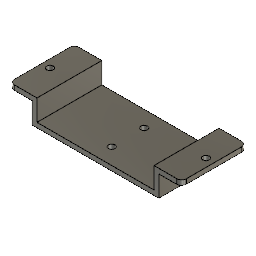
Chasis Quadra v19 (Autodesk Fusion 360 archive; units mm, degrees)
design "Soporte baterias"
Autodesk Fusion 360 part; units mm, degrees
sketch "Sketch1" plane through (0, 0, 0) normal (0, 0, 1) x (1, 0, 0)
  line L0 (0, 0) -> (78, 0)
  line L1 (78, 0) -> (78, 40)
  line L2 (78, 40) -> (0, 40)
  line L3 (0, 40) -> (0, 0)
  dimension "d1" = 78
  dimension "d2" = 40
  constraint horizontal L0
  constraint vertical L1
  constraint horizontal L2
  constraint vertical L3
  constraint coincident L0.start L3.end
  measures "d1" distance of L1.end L2.end
  measures "d2" distance of L0.start L2.end
extrude "Extrude1" add sketch "Sketch1" along normal blind 3
sketch "Sketch3" plane through (0, 0, 3) normal (0, 0, 1) x (-1, 0, 0)
  line L0 (0, -40) -> (0, 0)
  line L1 (0, 0) -> (-78, 0)
  line L2 (-78, 0) -> (-78, -40)
  line L3 (-78, -40) -> (0, -40)
  line L4 (0, -40) -> (-3, -40)
  line L5 (-3, -40) -> (-3, 0)
  line L6 (0, 0) -> (0, -40)
  dimension "d5" = 3
  constraint coincident L0.start L3.end
  constraint perpendicular L0 L4
  constraint coincident L1 L5.end
  constraint perpendicular L1 L5
  constraint coincident L0.end L1.start
  measures "d5" distance of L0.start L4.end
extrude "Extrude2" add sketch "Sketch3" along normal blind 13 contours L0 L1 L3 L4 L5 L6
sketch "Sketch4" plane through (0, 0, 3) normal (0, 0, 1) x (-1, 0, 0)
  line L0 (-3, -40) -> (-3, 0)
  line L1 (-3, 0) -> (-78, 0)
  line L2 (-78, 0) -> (-78, -40)
  line L3 (-78, -40) -> (-3, -40)
  line L4 (-78, -40) -> (-75, -40)
  line L5 (-75, -40) -> (-75, 0)
  line L6 (-78, 0) -> (-78, -40)
  dimension "d8" = 3
  constraint coincident L2.end L3.start
  constraint perpendicular L2 L4
  constraint coincident L1 L5.end
  constraint perpendicular L1 L5
  constraint coincident L1.end L2.start
  measures "d8" distance of L2.end L4.end
extrude "Extrude3" add sketch "Sketch4" along normal blind 13 contours L1 L2 L3 L4 L5 L6
sketch "Sketch5" plane through (78, 0, 0) normal (1, 0, 0) x (0, 1, 0)
  line L0 (0, 0) -> (40, 0)
  line L1 (40, 0) -> (40, 16)
  line L2 (40, 16) -> (0, 16)
  line L3 (0, 16) -> (0, 0)
  line L4 (40, 16) -> (40, 13)
  line L5 (40, 13) -> (0, 13)
  line L6 (0, 13) -> (0, 16)
  constraint coincident L1.end L2.start
  constraint coincident L1 L4.end
  constraint perpendicular L2 L4
  constraint coincident L3 L5.end
  constraint perpendicular L3 L5
  constraint coincident L2.end L3.start
  constraint perpendicular L2 L6
extrude "Extrude4" add sketch "Sketch5" along normal blind 14 contours L1 L2 L3 L4 L5 L6
sketch "Sketch6" plane through (0, 0, 0) normal (-1, 0, 0) x (0, -1, 0)
  line L0 (-40, 0) -> (0, 0)
  line L1 (0, 0) -> (0, 16)
  line L2 (0, 16) -> (-40, 16)
  line L3 (-40, 16) -> (-40, 0)
  line L4 (-40, 16) -> (0, 16)
  line L5 (0, 16) -> (0, 13)
  line L6 (0, 13) -> (-40, 13)
  line L7 (-40, 13) -> (-40, 16)
  constraint coincident L2.end L3.start
  constraint coincident L1.end L2.start
  constraint coincident L1 L5.end
  constraint perpendicular L4 L5
  constraint coincident L3 L6.end
  constraint perpendicular L3 L6
  constraint perpendicular L2 L7
extrude "Extrude5" add sketch "Sketch6" along normal blind 14 contours L1 L2 L3 L4 L5 L6 L7
sketch "Sketch7" plane through (0, 0, 16) normal (0, 0, 1) x (-1, 0, 0)
  line L0 (14, 0) -> (-3, 0)
  line L1 (-3, 0) -> (-3, -40)
  line L2 (-3, -40) -> (14, -40)
  line L3 (14, -40) -> (14, 0)
  circle A0 centre (9, -20) radius 2
  dimension "d15" = 4
  measures "d15" diameter of A0
extrude "Extrude6" cut sketch "Sketch7" against normal blind 3 contours A0
sketch "Sketch8" plane through (0, 0, 16) normal (0, 0, 1) x (-1, 0, 0)
  line L0 (-92, -40) -> (-75, -40)
  line L1 (-75, -40) -> (-75, 0)
  line L2 (-75, 0) -> (-92, 0)
  line L3 (-92, 0) -> (-92, -40)
  line L4 (-92, -20) -> (-87, -20)
  circle A0 centre (-87, -20) radius 2
  dimension "d18" = 4
  constraint midpoint L3 L4.start
  constraint perpendicular L3 L4
  constraint coincident L4.end A0.centre
  measures "d18" diameter of A0
extrude "Extrude7" cut sketch "Sketch8" against normal blind 3 contours A0
fillet "Fillet1" radius 3 1 edges at (-14, 0, 14.5)
fillet "Fillet2" radius 3 1 edges at (-14, 40, 14.5)
fillet "Fillet3" radius 3 1 edges at (92, 0, 14.5)
fillet "Fillet4" radius 3 1 edges at (92, 40, 14.5)
sketch "Sketch9" plane through (0, 0, 3) normal (0, 0, 1) x (-1, 0, 0)
  line L0 (-75, 0) -> (-75, -40)
  line L1 (-75, -40) -> (-3, -40)
  line L2 (-3, -40) -> (-3, 0)
  line L3 (-3, 0) -> (-75, 0)
  line L4 (-39, -40) -> (-39, 0)
  line L5 (-3, -20) -> (-75, -20)
  circle A0 centre (-39, -30) radius 2
  circle A1 centre (-39, -10) radius 2
  dimension "d25" = 4
  dimension "d26" = 4
  dimension "d27" = 10
  dimension "d28" = 10
  constraint midpoint L1 L4.start
  constraint midpoint L3 L4.end
  constraint midpoint L2 L5.start
  constraint midpoint L0 L5.end
  constraint coincident L4 A0.centre
  constraint coincident L4 A1.centre
  measures "d25" diameter of A0
  measures "d26" diameter of A1
  measures "d27" distance of L5 A0.centre
  measures "d28" distance of L5 A1.centre
extrude "Extrude8" cut sketch "Sketch9" against normal blind 3 contours L4 A1 | L4 A1 | L4 A0 | L4 A0
